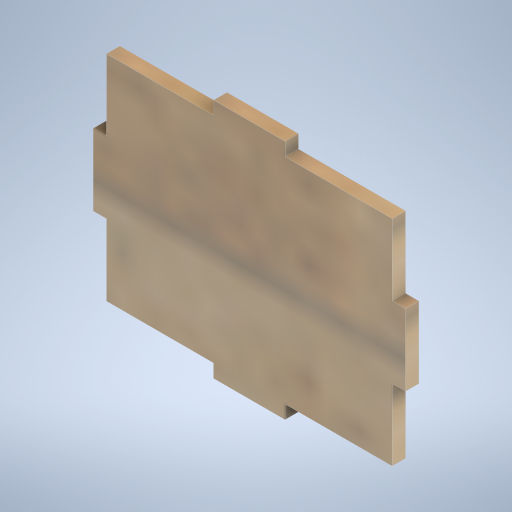
# Autodesk Inventor part: front plate
Saved by Autodesk Inventor 2023 (Build 270158000, 158)
## iProperties
Created: 2023-06-06
Part Number: front plate
Material: Hardboard
Document SubType Name: Sheet Metal
Designer: Ronan
Density: 0.799949 g/cm^3
Sheet Metal Rule: Default_mm
Appearance: Natural Maple - Glossy Dark Tint(1)
Author: Ronan
Autodesk Inventor part; units mm, degrees
ref_plane "YZ Plane" through (0, 0, 0) normal (1, 0, 0) x (0, 1, 0)
ref_plane "XZ Plane" through (0, 0, 0) normal (0, 1, 0) x (-1, 0, 0)
ref_plane "XY Plane" through (0, 0, 0) normal (0, 0, 1) x (1, 0, 0)
sketch "Sketch1" plane through (0, 0, 0) normal (0, 0, 1) x (1, 0, 0)
  line L0 (-24, 48) -> (-24, 51)
  line L1 (-24, 51) -> (-40, 51)
  line L2 (-40, 51) -> (-40, 48)
  line L3 (0, 32) -> (3, 32)
  line L4 (3, 32) -> (3, 16)
  line L5 (3, 16) -> (0, 16)
  line L6 (-40, 0) -> (-40, -3)
  line L7 (-40, -3) -> (-24, -3)
  line L8 (-24, -3) -> (-24, 0)
  line L9 (-64, 16) -> (-67, 16)
  line L10 (-67, 16) -> (-67, 32)
  line L11 (-67, 32) -> (-64, 32)
  line L12 (-64, 48) -> (-40, 48)
  line L13 (-24, 48) -> (0, 48)
  line L14 (-64, 0) -> (-64, 16)
  line L15 (-64, 32) -> (-64, 48)
  line L16 (0, 0) -> (-24, 0)
  line L17 (-40, 0) -> (-64, 0)
  line L18 (0, 48) -> (0, 32)
  line L19 (0, 16) -> (0, 0)
  point P0 (0, 0)
  dimension "d3" = 16
  dimension "d4" = 16
  dimension "d8" = 64
  dimension "d9" = 48
  dimension "d10" = 3
  dimension "d11" = 3
  dimension "d12" = 24
  dimension "d13" = 24
  dimension "d14" = 16
  dimension "d15" = 3
  measures "d3" distance of L0.end L1.end
  measures "d4" distance of L3.end L4.end
  measures "d8" distance between parallel lines of L18 L15
  measures "d9" distance between parallel lines of L17 L12
  measures "d10" distance of L10.end L11.end
  measures "d11" distance of L6.start L6.end
  measures "d12" distance of L0.start L13.end
  measures "d13" distance of L12.start L2.end
  measures "d14" distance of L6.end L7.end
  measures "d15" distance of L1.end L2.end
extrude "Plate1" add sketch "Sketch1" along normal blind 3
equation "\"d16\" = Thickness"
equation "\"BendRadius\" = Thickness"
equation "\"BendReliefWidth\" = Thickness"
equation "\"BendReliefDepth\" = 0.5 * Thickness"
equation "\"CornerReliefSize\" = 4 * Thickness"
equation "\"MinimumRemnant\" = 2 * Thickness"
equation "\"TransitionRadius\" = BendRadius"
equation "\"JacobiRadiusSize\" = BendRadius"
equation "\"GapSize\" = Thickness"
equation "\"Thickness\" = 3"
body "Solid1"
